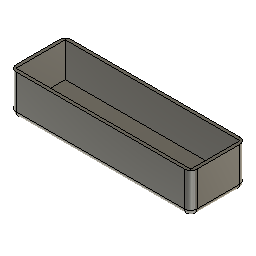
pilldaddy_buttoncover v1 (Autodesk Fusion 360 design; units mm, degrees)
Autodesk Fusion 360 part; units mm, degrees
sketch "Sketch1" plane through (0, 0, 0) normal (0, 0, 1) x (1, 0, 0)
  line L0 (-50, 25) -> (7.7, 25)
  line L1 (7.7, 25) -> (7.7, 7.3)
  line L2 (7.7, 7.3) -> (-50, 7.3)
  line L3 (-50, 7.3) -> (-50, 25)
  line L4 (6.7, 8.3) -> (-49, 8.3)
  line L5 (-49, 8.3) -> (-49, 24)
  line L6 (-49, 24) -> (6.7, 24)
  line L7 (6.7, 24) -> (6.7, 8.3)
  line L8 (6.7, 8.3) -> (-49, 24) construction
  line L9 (-49, 8.3) -> (6.7, 24) construction
  point P0 (-21.15, 16.15)
  dimension "d1" = 57.7
  dimension "d2" = 17.7
  dimension "d3" = 55.7
  dimension "d4" = 15.7
  constraint horizontal L0
  constraint vertical L1
  constraint horizontal L2
  constraint vertical L3
  constraint horizontal L4
  constraint perpendicular L4 L5
  constraint parallel L4 L6
  constraint parallel L5 L7
  constraint coincident L8 P0
  constraint coincident L9 P0
  measures "d1" distance of L0.start L0.end
  measures "d2" distance of L0.start L2.end
  measures "d3" distance of L5.end L6.end
  measures "d4" distance of L4.end L5.end
extrude "Extrude1" add sketch "Sketch1" along normal blind 2 contours L4 L5 L6 L7
extrude "Extrude2" add sketch "Sketch1" along normal blind 13
fillet "Fillet1" radius 2 4 edges at (7.7, 7.3, 6.5) (7.7, 25, 6.5) (-50, 7.3, 6.5) (-50, 25, 6.5)
fillet "Fillet2" radius 2 8 edges at (7.1142, 7.8858, 0) (-21.15, 7.3, 0) (-49.4142, 7.8858, 0) (-50, 16.15, 0) (-49.4142, 24.4142, 0) (-21.15, 25, 0) (7.1142, 24.4142, 0) (7.7, 16.15, 0)
